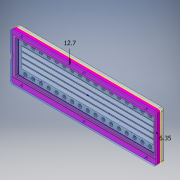
# Autodesk Inventor part: copy_stand_light
Saved by Autodesk Inventor 2019 (Build 230136000, 136)
## iProperties
Created: 2018-12-01
Part Number: copy_stand_light
Material: Generic
Document SubType Name: Modeling
Designer: caleb
Density: 1 g/cm^3
Appearance: Default
Author: caleb
Autodesk Inventor part; units mm, degrees
ref_plane "YZ Plane" through (0, 0, 0) normal (1, 0, 0) x (0, 1, 0)
ref_plane "XZ Plane" through (0, 0, 0) normal (0, 1, 0) x (-1, 0, 0)
sketch "Sketch1" plane through (0, 0, 0) normal (0, 0, 1) x (1, 0, 0)
  line L0 (-139.7, 0) -> (139.7, 0)
  line L1 (139.7, 0) -> (139.7, 90.8)
  line L2 (139.7, 90.8) -> (-139.7, 90.8)
  line L3 (-139.7, 90.8) -> (-139.7, 0)
  line L4 (-139.7, 0) -> (139.7, 90.8) construction
  line L5 (139.7, 0) -> (-139.7, 90.8) construction
  point P0 (0, 0)
  point P1 (0, 45.4)
  point P2 (0, 0)
  dimension "d0" = 279.4
  dimension "d1" = 90.8
  constraints: 12 end point, 3 midpoint, 2 parallel, 1 coincident, 1 horizontal, 1 perpendicular
  measures "d0" distance of L0.start L0.end
  measures "d1" distance of L0.end L1.end
extrude "Extrusion1" add sketch "Sketch1" along normal blind 6.35
fillet "Fillet1" radius 4 4 edges at (139.7, 0, 3.175) (139.7, 90.8, 3.175) (-139.7, 90.8, 3.175) (-139.7, 0, 3.175)
sketch "Sketch2" plane through (0, 0, 6.35) normal (0, 0, 1) x (1, 0, 0)
  line L0 (-127, 56.4) -> (127, 56.4)
  line L1 (127, 56.4) -> (127, 64.4)
  line L2 (127, 64.4) -> (-127, 64.4)
  line L3 (-127, 64.4) -> (-127, 56.4)
  line L4 (-127, 56.4) -> (127, 64.4) construction
  line L5 (127, 56.4) -> (-127, 64.4) construction
  line L6 (-139.7, 90.8) -> (-139.7, 0) projected
  point P0 (0, 0)
  point P1 (0, 60.4)
  point P2 (0, 60.4)
  point P3 (0, 60.4)
  point P4 (-139.7, 45.4)
  dimension "d4" = 254
  dimension "d5" = 8
  dimension "d15" = 90.8
  dimension "d17" = 15
  constraints: 12 end point, 5 midpoint, 2 parallel, 1 horizontal, 1 perpendicular, 1 vertical alignment
  measures "d4" distance of L0.start L0.end
  measures "d5" distance of L0.end L1.end
  measures "d15" distance of L6.start L6.end
  measures "d17" vertical distance of point (0, 60.4) point (-139.7, 45.4)
extrude "Extrusion2" add sketch "Sketch2" along normal blind 0.5 separate body
pattern_linear "Rectangular Pattern1" count 4 spacing 10 along (0, -1, 0) bodies 2
sketch "Sketch3" plane through (0, 0, 6.35) normal (0, 0, 1) x (1, 0, 0)
  line L0 (-135.7, 0) -> (135.7, 0) projected
  line L1 (139.7, 4) -> (139.7, 86.8) projected
  line L2 (135.7, 90.8) -> (-135.7, 90.8) projected
  line L3 (-139.7, 86.8) -> (-139.7, 4) projected
  arc A0 (-139.7, 4) -> (-135.7, 0) centre (-135.7, 4) ccw projected
  arc A1 (135.7, 0) -> (139.7, 4) centre (135.7, 4) ccw projected
  arc A2 (139.7, 86.8) -> (135.7, 90.8) centre (135.7, 86.8) ccw projected
  arc A3 (-135.7, 90.8) -> (-139.7, 86.8) centre (-135.7, 86.8) ccw projected
  line L4 (-133.35, 12.7) -> (133.35, 12.7)
  line L5 (133.35, 12.7) -> (133.35, 78.1)
  line L6 (133.35, 78.1) -> (-133.35, 78.1)
  line L7 (-133.35, 78.1) -> (-133.35, 12.7)
  line L8 (-133.35, 12.7) -> (133.35, 78.1) construction
  line L9 (133.35, 12.7) -> (-133.35, 78.1) construction
  point P0 (0, 0)
  point P1 (0, 45.4)
  point P2 (0, 0)
  point P3 (0, 45.4)
  point P4 (0, 45.4)
  point P5 (-139.7, 45.4)
  dimension "d32" = 6.35
  dimension "d33" = 12.7
  constraints: 12 end point, 6 midpoint, 2 parallel, 1 horizontal, 1 horizontal alignment, 1 perpendicular, 1 vertical alignment
  measures "d32" distance between parallel lines of L1 L5
  measures "d33" distance between parallel lines of L2 L6
extrude "Extrusion3" add sketch "Sketch3" along normal blind 6.35 separate body
fillet "Fillet2" radius 2 4 edges at (-133.35, 78.1, 9.525) (-133.35, 12.7, 9.525) (133.35, 12.7, 9.525) (133.35, 78.1, 9.525)
sketch "Sketch4" plane through (0, 0, 6.35) normal (0, 0, 1) x (1, 0, 0)
  line L0 (-135.7, 0) -> (135.7, 0) construction
  line L1 (139.7, 4) -> (139.7, 86.8) construction
  line L2 (135.7, 90.8) -> (-135.7, 90.8) construction
  line L3 (-139.7, 86.8) -> (-139.7, 4) construction
  line L4 (139.7, 90.8) -> (-139.7, 90.8) construction
  line L5 (0, 90.8) -> (0, 0) construction
  line L6 (127, 64.4) -> (-127, 64.4) construction
  arc A0 (-139.7, 4) -> (-135.7, 0) centre (-135.7, 4) ccw projected
  arc A1 (135.7, 0) -> (139.7, 4) centre (135.7, 4) ccw projected
  arc A2 (139.7, 86.8) -> (135.7, 90.8) centre (135.7, 86.8) ccw projected
  arc A3 (-135.7, 90.8) -> (-139.7, 86.8) centre (-135.7, 86.8) ccw projected
  line L7 (0, 78.1) -> (0, 64.4) construction
  line L8 (-131.35, 78.1) -> (131.35, 78.1) projected
  point P0 (0, 71.25)
  constraints: 4 end point, 4 midpoint, 1 point on line, 1 vertical
hole "Hole1" at (0, 71.25, 6.35) direction (0, 0, -1) diameter 6.756 end through all bodies 1 clearance for "Flat Head Machine Screw (82)" size "1/4" standard "Ansi Unified Screw Threads"
pattern_linear "Rectangular Pattern2" count 17 spacing 15 along (1, 0, 0) of "Hole1" first direction both ways yes bodies 1
ref_plane "Work Plane1" through (-139.7, 45.4, 0) normal (0, -1, 0) x (1, 0, 0)
mirror "Mirror1" about plane through (-139.7, 45.4, 0) normal (0, -1, 0) of "Hole1", "Rectangular Pattern2" bodies 1
sketch "Sketch7" plane through (0, 0, 12.7) normal (0, 0, 1) x (1, 0, 0)
  line L0 (-133.35, 14.7) -> (-133.35, 76.1) projected
  arc A0 (-131.35, 78.1) -> (-133.35, 76.1) centre (-131.35, 76.1) ccw projected
  line L1 (-131.35, 78.1) -> (131.35, 78.1) projected
  arc A1 (133.35, 76.1) -> (131.35, 78.1) centre (131.35, 76.1) ccw projected
  line L2 (133.35, 76.1) -> (133.35, 14.7) projected
  arc A2 (131.35, 12.7) -> (133.35, 14.7) centre (131.35, 14.7) ccw projected
  line L3 (131.35, 12.7) -> (-131.35, 12.7) projected
  arc A3 (-133.35, 14.7) -> (-131.35, 12.7) centre (-131.35, 14.7) ccw projected
  arc A4 (-139.7, 4) -> (-135.7, 0) centre (-135.7, 4) ccw projected
  line L4 (-135.7, 0) -> (135.7, 0) projected
  arc A5 (135.7, 0) -> (139.7, 4) centre (135.7, 4) ccw projected
  line L5 (139.7, 4) -> (139.7, 86.8) projected
  arc A6 (139.7, 86.8) -> (135.7, 90.8) centre (135.7, 86.8) ccw projected
  line L6 (135.7, 90.8) -> (-135.7, 90.8) projected
  arc A7 (-135.7, 90.8) -> (-139.7, 86.8) centre (-135.7, 86.8) ccw projected
  line L7 (-139.7, 86.8) -> (-139.7, 4) projected
  point P0 (0, 0)
sketch "Sketch6" plane through (0, 0, 12.7) normal (0, 0, 1) x (1, 0, 0)
  line L0 (-136.35, 9.7) -> (136.35, 9.7)
  line L1 (136.35, 9.7) -> (136.35, 81.1)
  line L2 (136.35, 81.1) -> (-136.35, 81.1)
  line L3 (-136.35, 81.1) -> (-136.35, 9.7) construction
  line L4 (-136.35, 9.7) -> (136.35, 81.1) construction
  line L5 (136.35, 9.7) -> (-136.35, 81.1) construction
  line L6 (-135.7, 0) -> (135.7, 0) projected
  line L7 (-133.35, 14.7) -> (-133.35, 76.1) projected
  line L8 (131.35, 12.7) -> (-131.35, 12.7) projected
  line L9 (-136.35, 81.1) -> (136.35, 81.1) construction
  line L10 (-136.35, 81.1) -> (-139.7, 81.1)
  line L11 (-139.7, 81.1) -> (-139.7, 9.7)
  line L12 (-139.7, 9.7) -> (-136.35, 9.7)
  line L13 (-136.35, 9.7) -> (-136.35, 81.1) construction
  line L14 (-139.7, 86.8) -> (-139.7, 4) projected
  point P0 (0, 0)
  point P1 (0, 45.4)
  dimension "d36" = 3
  dimension "d37" = 3
  constraints: 22 end point, 4 parallel, 3 horizontal, 2 midpoint, 2 perpendicular, 1 point on line
  measures "d36" distance between parallel lines of L7 L3
  measures "d37" distance between parallel lines of L0 L8
extrude "Extrusion5" cut sketch "Sketch6" against normal blind 0.5 bodies 3
extrude "Extrusion6" add sketch "Sketch7" along normal blind 3.175 separate body contours L0 A0 L1 A1 L2 A2 L3 A3 | L7 A7 L6 A6 L5 A5 L4 A4
sketch "Sketch8" plane through (0, 0, 15.875) normal (0, 0, 1) x (1, 0, 0)
  arc A0 (-139.7, 4) -> (-135.7, 0) centre (-135.7, 4) ccw construction
  line L0 (-135.7, 0) -> (135.7, 0) construction
  arc A1 (135.7, 0) -> (139.7, 4) centre (135.7, 4) ccw construction
  line L1 (139.7, 4) -> (139.7, 86.8) construction
  arc A2 (139.7, 86.8) -> (135.7, 90.8) centre (135.7, 86.8) ccw construction
  line L2 (135.7, 90.8) -> (-135.7, 90.8) construction
  arc A3 (-135.7, 90.8) -> (-139.7, 86.8) centre (-135.7, 86.8) ccw construction
  line L3 (-139.7, 86.8) -> (-139.7, 4) construction
  line L4 (135.7, 90.8) -> (-135.7, 90.8) projected
  line L5 (0, 90.8) -> (0, 81.1)
  line L6 (-139.7, 81.1) -> (136.35, 81.1) projected
  point P0 (0, 0)
  point P1 (0, 85.95)
  point P2 (0, 45.4)
  point P3 (0, 85.95)
  constraints: 2 end point, 2 midpoint, 1 coincident, 1 point on line, 1 vertical alignment
hole "Hole3" at (0, 85.95, 15.875) direction (0, 0, -1) diameter 3.264 end through all bodies 4 3 1 clearance for "Flat Head Machine Screw (82)" size "#4" standard "Ansi Unified Screw Threads"
pattern_linear "Rectangular Pattern3" count 3 spacing 120 along (-1, 0, 0) of "Hole3" first direction both ways yes bodies 4 3 1
mirror "Mirror2" about plane through (-139.7, 45.4, 0) normal (0, -1, 0) of "Hole3", "Rectangular Pattern3" bodies 1 3 4
sketch "Sketch10" plane through (0, 0, 12.2) normal (0, 0, 1) x (1, 0, 0)
  arc A0 (133.35, 76.1) -> (131.35, 78.1) centre (131.35, 76.1) ccw projected
  line L0 (133.35, 14.7) -> (133.35, 76.1) projected
  arc A1 (131.35, 12.7) -> (133.35, 14.7) centre (131.35, 14.7) ccw projected
  line L1 (-131.35, 12.7) -> (131.35, 12.7) projected
  arc A2 (-133.35, 14.7) -> (-131.35, 12.7) centre (-131.35, 14.7) ccw projected
  line L2 (-133.35, 76.1) -> (-133.35, 14.7) projected
  arc A3 (-131.35, 78.1) -> (-133.35, 76.1) centre (-131.35, 76.1) ccw projected
  line L3 (131.35, 78.1) -> (-131.35, 78.1) projected
  line L4 (136.35, 9.7) -> (-139.7, 9.7) projected
  line L5 (136.35, 81.1) -> (136.35, 9.7) projected
  line L6 (-139.7, 81.1) -> (136.35, 81.1) projected
  line L7 (-139.7, 9.7) -> (-139.7, 81.1) projected
  line L8 (135.85, 80.6) -> (135.85, 10.2)
  line L9 (135.85, 10.2) -> (-139.2, 10.2)
  line L10 (-139.2, 10.2) -> (-139.2, 80.6)
  line L11 (-139.2, 80.6) -> (135.85, 80.6)
  point P0 (0, 0)
  dimension "d59" = 0.5
  constraints: 8 end point, 3 other
  measures "d59" distance between parallel lines of L6 L11
extrude "Extrusion7" add sketch "Sketch10" along normal blind 0.1 separate body contours L0 A1 L1 A2 L2 A3 L3 A0 | L8 L9 L10 L11
sketch "Sketch11" plane through (0, 0, 6.35) normal (0, 0, 1) x (1, 0, 0)
  line L0 (-127, 56.4) -> (127, 56.4) projected
  line L1 (127, 56.4) -> (127, 64.4) projected
  line L2 (127, 64.4) -> (-127, 64.4) projected
  line L3 (-127, 64.4) -> (-127, 56.4) projected
  line L4 (-127, 46.4) -> (127, 46.4) projected
  line L5 (127, 46.4) -> (127, 54.4) projected
  line L6 (127, 54.4) -> (-127, 54.4) projected
  line L7 (-127, 54.4) -> (-127, 46.4) projected
  line L8 (-127, 36.4) -> (127, 36.4) projected
  line L9 (127, 36.4) -> (127, 44.4) projected
  line L10 (127, 44.4) -> (-127, 44.4) projected
  line L11 (-127, 44.4) -> (-127, 36.4) projected
  line L12 (-127, 26.4) -> (127, 26.4) projected
  line L13 (127, 26.4) -> (127, 34.4) projected
  line L14 (127, 34.4) -> (-127, 34.4) projected
  line L15 (-127, 34.4) -> (-127, 26.4) projected
  point P0 (0, 0)
extrude "Extrusion8" cut sketch "Sketch11" against normal blind 0.1 bodies 1
sketch "Sketch12" plane through (0, 0, 15.875) normal (0, 0, 1) x (1, 0, 0)
  circle A0 centre (-145.7, 45.4) radius 9
  line L0 (-139.7, 86.8) -> (-139.7, 4) projected
  point P0 (0, 0)
  point P1 (0, 45.4)
  dimension "d64" = 6
  dimension "d65" = 18
  constraints: 1 centre point, 1 horizontal alignment
  measures "d64" horizontal distance of A0.centre L0.end
  measures "d65" diameter of A0
extrude "Extrusion9" cut sketch "Sketch12" against normal through all bodies 4
equation "\"d2\" = thickness"
equation "\"d13\" = thickness"
equation "\"d65\" = 3 * d64"
equation "\"thickness\" = 6.35"
